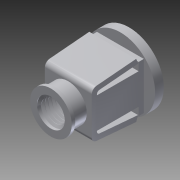
# Autodesk Inventor part: Screw housing
Saved by Autodesk Inventor 2014 SP2 (Build 180246200, 246)
## iProperties
Created: 2015-10-09
Part Number: Screw housing
Material: PC/ABS Plastic
Document SubType Name: Modeling
Designer: Lukasz Szmit
Density: 0.357273 g/cm^3
Appearance: Smooth - White
Author: Lukasz Szmit
Autodesk Inventor part; units mm, degrees
sketch "Sketch1" plane through (0, 0, 0) normal (0, 1, 0) x (-1, 0, 0)
  circle A0 centre (0, 0) radius 10
  dimension "d13" = 20
  constraints: 1 centre point, 1 coincident
  measures "d13" diameter of A0
extrude "Extrusion1" add sketch "Sketch1" against normal blind 2.5
sketch "Sketch2" plane through (0, -2.5, 0) normal (0, -1, 0) x (1, 0, 0)
  circle A0 centre (0, 0) radius 10 construction
  line L0 (6.75, -6.75) -> (-6.75, -6.75)
  line L1 (-6.75, -6.75) -> (-6.75, 6.75)
  line L2 (-6.75, 6.75) -> (6.75, 6.75)
  line L3 (6.75, 6.75) -> (6.75, -6.75)
  line L4 (6.75, -6.75) -> (-6.75, 6.75) construction
  line L5 (-6.75, -6.75) -> (6.75, 6.75) construction
  dimension "d11" = 13.5
  dimension "d12" = 13.5
  constraints: 12 end point, 2 midpoint, 2 perpendicular, 1 parallel
  measures "d11" distance of L1.end L2.end
  measures "d12" distance of L2.end L0.start
extrude "Extrusion2" add sketch "Sketch2" along normal blind 15
sketch "Sketch12" plane through (0, -17.5, 0) normal (0, -1, 0) x (1, 0, 0)
  line L0 (6.75, -6.75) -> (6.75, 6.75) construction
  line L1 (-6.75, 6.75) -> (-6.75, -6.75) construction
  line L2 (-6.75, 6.75) -> (6.75, 6.75)
  line L3 (6.75, 6.75) -> (6.75, 4.425)
  line L4 (6.75, 4.425) -> (-6.75, 4.425)
  line L5 (-6.75, 4.425) -> (-6.75, 6.75)
  line L6 (-6.75, -4.425) -> (6.75, -4.425)
  line L7 (6.75, -4.425) -> (6.75, -6.75)
  line L8 (6.75, -6.75) -> (-6.75, -6.75)
  line L9 (-6.75, -6.75) -> (-6.75, -4.425)
  point P0 (0, 0)
  dimension "d32" = 13.5
  dimension "d33" = 2.325
  dimension "d34" = 2.325
  dimension "d35" = 13.5
  dimension "d36" = 4.425
  dimension "d37" = 4.425
  constraints: 16 end point, 2 point on line
  measures "d32" distance of L1.start L2.end
  measures "d33" distance of L3.end L0.end
  measures "d34" distance of L0.start L6.end
  measures "d35" distance of L0.start L1.end
  measures "d36" distance from line of point (0, 0) L4
  measures "d37" distance from line of point (0, 0) L6
extrude "Extrusion9" cut sketch "Sketch12" against normal blind 13.5
sketch "Sketch13" plane through (0, -17.5, 0) normal (0, -1, 0) x (1, 0, 0)
  line L0 (-6.75, -4.425) -> (6.75, -4.425) projected
  line L1 (6.75, -4.425) -> (6.75, 4.425) projected
  line L2 (6.75, 4.425) -> (-6.75, 4.425) projected
  line L3 (-6.75, 4.425) -> (-6.75, -4.425) projected
  line L4 (6.75, -6.75) -> (-6.75, -6.75)
  line L5 (-6.75, -6.75) -> (-6.75, 6.75)
  line L6 (-6.75, 6.75) -> (6.75, 6.75)
  line L7 (6.75, 6.75) -> (6.75, -6.75)
  line L8 (6.75, -6.75) -> (-6.75, 6.75) construction
  line L9 (-6.75, -6.75) -> (6.75, 6.75) construction
  point P0 (0, 0)
  dimension "d40" = 13.5
  dimension "d41" = 13.5
  constraints: 12 end point, 2 midpoint, 2 parallel, 1 perpendicular
  measures "d40" distance of L5.end L6.end
  measures "d41" distance of L4.end L5.end
extrude "Extrusion10" add sketch "Sketch13" against normal blind 1.5 contours L0 L7 L4 L5 | L5 L6 L7 L2
ref_plane "Work Plane9" through (-6.75, -17.5, 6.75) normal (0, -0.0871557, 0.9961947) x (1, 0, 0)
sketch "Sketch14" plane through (-6.75, -17.5, 6.75) normal (0, -0.0871557, 0.9961947) x (1, 0, 0)
  line L0 (0, 0) -> (13.5, 0) construction
  line L1 (13.5, 0) -> (13.5, 1.4943) construction
  line L2 (0, 1.4943) -> (13.5, 1.4943) construction
  line L3 (0, 0) -> (0, 1.4943) construction
  line L4 (0, 13.4486) -> (13.5, 13.4486) construction
  line L5 (13.5, 14.9429) -> (13.5, 13.4486) construction
  line L6 (0, 14.9429) -> (13.5, 14.9429) construction
  line L7 (0, 14.9429) -> (0, 13.4486) construction
  line L8 (13.5, 0) -> (0, 0)
  line L9 (0, 0) -> (0, 13.25)
  line L10 (0, 13.25) -> (13.5, 13.25)
  line L11 (13.5, 13.25) -> (13.5, 0)
  point P0 (6.75, 16.8451)
  dimension "d46" = 13.25
  dimension "d47" = 13.5
  constraints: 8 end point, 1 parallel, 1 perpendicular
  measures "d46" distance of L8.end L9.end
  measures "d47" distance of L9.end L10.end
extrude "Extrusion11" add sketch "Sketch14" against normal blind 1.5
fillet "Fillet2" radius 0.75 1 edges at (0, -16, 5.3755)
fillet "Fillet3" radius 1.5 1 edges at (0, -17.5, 6.75)
ref_plane "Work Plane10" through (6.75, -17.5, -6.75) normal (0, -0.0871557, -0.9961947) x (-1, 0, 0)
sketch "Sketch15" plane through (6.75, -17.5, -6.75) normal (0, -0.0871557, -0.9961947) x (-1, 0, 0)
  line L0 (0, 0) -> (13.5, 0) construction
  line L1 (13.5, 0) -> (13.5, 1.4943) construction
  line L2 (0, 1.4943) -> (13.5, 1.4943) construction
  line L3 (0, 0) -> (0, 1.4943) construction
  line L4 (0, 13.4486) -> (13.5, 13.4486) construction
  line L5 (13.5, 14.9429) -> (13.5, 13.4486) construction
  line L6 (0, 14.9429) -> (13.5, 14.9429) construction
  line L7 (0, 14.9429) -> (0, 13.4486) construction
  line L8 (13.5, 0) -> (0, 0)
  line L9 (0, 0) -> (0, 13.25)
  line L10 (0, 13.25) -> (13.5, 13.25)
  line L11 (13.5, 13.25) -> (13.5, 0)
  point P0 (6.75, 16.8451)
  dimension "d53" = 13.25
  dimension "d54" = 13.5
  constraints: 8 end point, 2 perpendicular, 1 parallel
  measures "d53" distance of L10.end L0.end
  measures "d54" distance of L9.end L10.end
extrude "Extrusion12" add sketch "Sketch15" against normal blind 1.5
fillet "Fillet4" radius 0.75 1 edges at (0, -16, -5.3755)
fillet "Fillet5" radius 1.5 1 edges at (0, -17.5, -6.75)
ref_plane "Work Plane11" through (6.75, -4.1697, -6.4105) normal (0, 0.9396926, -0.3420201) x (-1, 0, 0)
sketch "Sketch16" plane through (6.75, -4.1697, -6.4105) normal (0, 0.9396926, -0.3420201) x (-1, 0, 0)
  line L0 (0, -1.5529) -> (0, 0) construction
  line L1 (0, 0) -> (13.5, 0) construction
  line L2 (13.5, 0) -> (13.5, -1.5529) construction
  line L3 (13.5, -1.5529) -> (0, -1.5529) construction
  ellipse E0 centre (6.75, 6.8219) end of major axis (6.75, 17.4637) minor radius 10 (16.5824, 4.8818) -> (15.3838, 12.1913) ccw construction
  line L4 (16.5824, 4.8818) -> (13.5, 4.8818) construction
  line L5 (13.5, 4.8818) -> (13.5, 0.4961) construction
  line L6 (13.5, 0.4961) -> (0, 0.4961) construction
  line L7 (0, 0.4961) -> (0, 4.8818) construction
  line L8 (0, 4.8818) -> (-3.0824, 4.8818) construction
  ellipse E1 centre (6.75, 6.8219) end of major axis (6.75, 17.4637) minor radius 10 (-1.8838, 12.1913) -> (-3.0824, 4.8818) ccw construction
  line L9 (-1.8838, 12.1913) -> (15.3838, 12.1913) construction
  line L10 (13.5, -1.5529) -> (0, -1.5529)
  line L11 (0, -1.5529) -> (0, 0)
  line L12 (0, 0) -> (13.5, 0)
  line L13 (13.5, 0) -> (13.5, -1.5529)
  point P0 (6.75, 7.45)
  constraints: 8 end point, 2 other
revolve "Revolution1" cut sketch "Sketch16" angle 15 about axis through (6.75, -4.1697, -6.4105) along (1, 0, 0)
ref_plane "Work Plane12" through (-6.75, -4.1697, 6.4105) normal (0, 0.9396926, 0.3420201) x (1, 0, 0)
sketch "Sketch17" plane through (-6.75, -4.1697, 6.4105) normal (0, 0.9396926, 0.3420201) x (1, 0, 0)
  line L0 (13.5, 0) -> (13.5, -1.5529) construction
  line L1 (13.5, -1.5529) -> (0, -1.5529) construction
  line L2 (0, -1.5529) -> (0, 0) construction
  line L3 (0, 0) -> (13.5, 0) construction
  ellipse E0 centre (6.75, 6.8219) end of major axis (6.75, -3.8198) minor radius 10 (-1.8838, 12.1913) -> (-3.0824, 4.8818) ccw construction
  line L4 (-1.8838, 12.1913) -> (15.3838, 12.1913) construction
  ellipse E1 centre (6.75, 6.8219) end of major axis (6.75, -3.8198) minor radius 10 (16.5824, 4.8818) -> (15.3838, 12.1913) ccw construction
  line L5 (16.5824, 4.8818) -> (13.5, 4.8818) construction
  line L6 (13.5, 4.8818) -> (13.5, 0.4961) construction
  line L7 (13.5, 0.4961) -> (0, 0.4961) construction
  line L8 (0, 0.4961) -> (0, 4.8818) construction
  line L9 (0, 4.8818) -> (-3.0824, 4.8818) construction
  line L10 (13.5, -1.5529) -> (0, -1.5529)
  line L11 (0, -1.5529) -> (0, 0)
  line L12 (0, 0) -> (13.5, 0)
  line L13 (13.5, 0) -> (13.5, -1.5529)
  point P0 (6.75, 7.45)
  constraints: 8 end point, 2 other
revolve "Revolution2" cut sketch "Sketch17" angle 15 about axis through (-6.75, -4.1697, 6.4105) along (-1, 0, 0)
sketch "Sketch18" plane through (0, 0, 0) normal (0, 1, 0) x (1, 0, 0)
  circle A0 centre (0, 0) radius 10 projected
  constraints: 1 coincident
hole "Hole1" at (0, 0, 0) direction (0, -1, 0) diameter 8 end through all
ref_plane "Work Plane13" through (6.75, -4, 0) normal (0, 0, -1) x (-1, 0, 0)
sketch "Sketch19" plane through (6.75, -4, 0) normal (0, 0, -1) x (-1, 0, 0)
  line L0 (-3.25, 1.5) -> (-3.25, 4) construction
  line L1 (-3.25, 4) -> (2.75, 4) construction
  line L2 (2.75, 4) -> (2.75, -13.5) construction
  line L3 (2.75, -13.5) -> (0, -13.5) construction
  line L4 (0, -13.5) -> (0, 1.5) construction
  line L5 (0, 1.5) -> (-3.25, 1.5) construction
  line L6 (16.75, 4) -> (16.75, 1.5) construction
  line L7 (16.75, 1.5) -> (13.5, 1.5) construction
  line L8 (13.5, 1.5) -> (13.5, -13.5) construction
  line L9 (13.5, -13.5) -> (10.75, -13.5) construction
  line L10 (10.75, -13.5) -> (10.75, 4) construction
  line L11 (10.75, 4) -> (16.75, 4) construction
  line L12 (3.4909, 3.5005) -> (2.75, 3.0727)
  line L13 (3.491, 3.5722) -> (3.4909, 3.5005)
  line L14 (2.75, 3.0727) -> (2.75, 4)
  line L15 (3.491, 3.5722) -> (2.75, 4)
  line L16 (4, -58) -> (-4, -58)
  line L17 (6.75, 4) -> (6.75, -14.3748)
  point P0 (0, 0)
  dimension "d71" = 0.7409
  dimension "d72" = 60
  dimension "d73" = 0.0717
  constraints: 12 end point
  measures "d71" horizontal distance of L12.start L12.end
  measures "d72" angle of L12 L15
  measures "d73" distance of L13.start L12.start
coil "Coil1" sketch "Sketch19" operation add axis through (0, -10, 0) along (0, -1, 0) pitch 1 turns 21.5 hand right
sketch "Sketch20" plane through (0, -17.5, 0) normal (0, -1, 0) x (1, 0, 0)
  circle A0 centre (0, 0) radius 4 projected
  circle A1 centre (0, 0) radius 5.325
  circle A2 centre (0, 0) radius 4
  constraints: 2 centre point, 2 coincident
extrude "Extrusion13" add sketch "Sketch20" along normal blind 5
sketch "Sketch21" plane through (0, -22.5, 0) normal (0, -1, 0) x (1, 0, 0)
  circle A0 centre (0, 0) radius 5.325 projected
  circle A1 centre (0, 0) radius 6
  constraints: 1 centre point, 1 coincident
extrude "Extrusion14" add sketch "Sketch21" against normal blind 1
equation "\"d12\" = d11"
equation "\"d37\" = d36"
equation "\"d41\" = d40"
body "Solid1"
